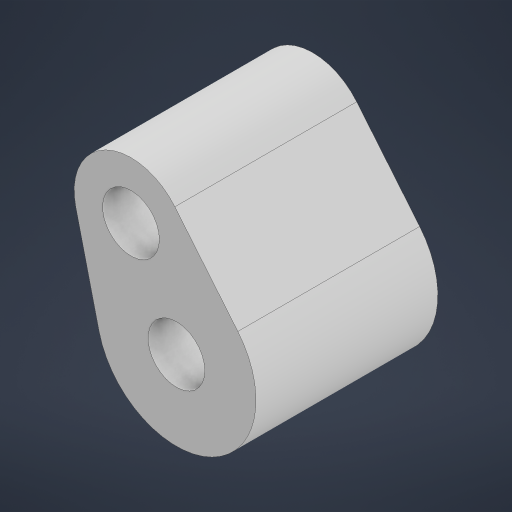
# Autodesk Inventor part: pto
Saved by Autodesk Inventor 2024 (Build 280153000, 153)
## iProperties
Created: 2023-11-19
Part Number: pto
Material: Generic
Document SubType Name: Modeling
Designer: macbook
Density: 1 g/cm^3
Appearance: Default
Author: macbook
Autodesk Inventor part; units mm, degrees
ref_plane "YZ Plane" through (0, 0, 0) normal (1, 0, 0) x (0, 1, 0)
ref_plane "XZ Plane" through (0, 0, 0) normal (0, 1, 0) x (-1, 0, 0)
ref_plane "XY Plane" through (0, 0, 0) normal (0, 0, 1) x (1, 0, 0)
sketch "Sketch1" plane through (0, 0, 0) normal (0, 0, 1) x (1, 0, 0)
  line L0 (0, 0) -> (0, -12.7)
  line L1 (0, -12.7) -> (6.35, -12.7)
  circle A0 centre (0, 0) radius 3.9688
  circle A1 centre (6.35, -12.7) radius 3.9687
  circle A2 centre (0, 0) radius 7.9375
  circle A3 centre (6.35, -12.7) radius 11.1125
  line L2 (0, 0) -> (6.35, -12.7)
  line L3 (0, 0) -> (-7.0995, -3.5498)
  line L4 (6.35, -12.7) -> (-3.5893, -17.6697)
  line L5 (-9.9727, 7.4348) -> (-2.1627, -24.7395)
  line L6 (-1.2787, 14.0345) -> (19.7747, -11.518)
  point P0 (7.7583, -1.6771)
  point P1 (-7.7135, -1.8724)
  point P2 (-4.4489, -15.3213)
  point P3 (14.9264, -5.6337)
  point P4 (6.126, 5.0474)
  dimension "d4" = 15.875
  dimension "d5" = 22.225
  dimension "d0" = 12.7
  dimension "d1" = 6.35
  dimension "d2" = 7.9375
  dimension "d3" = 7.9375
  constraints: 14 end point, 4 coincident, 2 centre point, 1 horizontal, 1 parallel, 1 vertical, 10 other
  measures "d0" distance of L0.start L0.end
  measures "d1" distance of L0.end L1.end
  measures "d2" diameter of A0
  measures "d3" diameter of A1
extrude "Extrusion1" add sketch "Sketch1" along normal blind 25.4 contours L3 A2 A3 A0 | A0 A3 A2 L3 | A0 L2 A2 L0 | L0 A2 A3 A0 | A3 A2 L2 A0 | A2 A3 L5 | A2 L2 A1 L1 L0 | L0 L1 A1 L4 A3 A2 | A3 L4 A1 L2 A2 | A2 L6 A3
body "Solid1"
